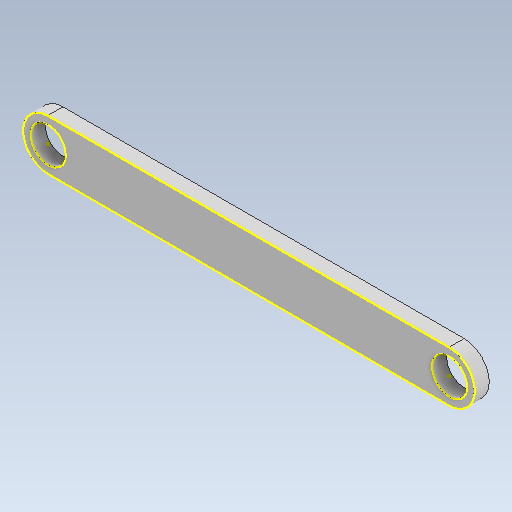
# Autodesk Inventor part: adjustable_80
Saved by Autodesk Inventor 2023 (Build 270158000, 158)
## iProperties
Created: 2023-04-16
Part Number: adjustable_80
Material: 一般
Document SubType Name: Modeling
Designer: JOU
Density: 1 g/cm^3
Appearance: 預設
Author: JOU
Autodesk Inventor part; units mm, degrees
ref_plane "YZ Plane" through (0, 0, 0) normal (1, 0, 0) x (0, 1, 0)
ref_plane "XZ Plane" through (0, 0, 0) normal (0, 1, 0) x (-1, 0, 0)
ref_plane "XY Plane" through (0, 0, 0) normal (0, 0, 1) x (1, 0, 0)
sketch "草圖1" plane through (0, 0, 0) normal (0, 0, 1) x (1, 0, 0)
  line L0 (-80, 0) -> (0, 0) construction
  line L1 (-80, -5) -> (0, -5)
  line L2 (0, 5) -> (-80, 5)
  arc A0 (-80, 5) -> (-80, -5) centre (-80, 0) ccw
  arc A1 (0, -5) -> (0, 5) centre (0, 0) ccw
  circle A2 centre (-80, 0) radius 3.5
  circle A3 centre (0, 0) radius 3.5
  point P0 (-40, 0)
  dimension "d0" = 80
  dimension "d1" = 10
  dimension "d2" = 7
  dimension "d3" = 7
  constraints: 8 end point, 4 centre point, 4 point on circle, 4 tangent, 3 coincident, 1 horizontal, 1 midpoint, 1 parallel
  measures "d0" distance of L2.start L2.end
  measures "d1" distance between parallel lines of L1 L2
  measures "d2" diameter of A2
  measures "d3" diameter of A3
extrude "擠出1" add sketch "草圖1" along normal blind 3
sketch "草圖5" plane through (0, 0, 3) normal (0, 0, 1) x (1, 0, 0)
  arc A0 (0, -5) -> (0, 5) centre (0, 0) ccw projected
  line L0 (0, 5) -> (-80, 5) projected
  arc A1 (-80, 5) -> (-80, -5) centre (-80, 0) ccw projected
  line L1 (-80, -5) -> (0, -5) projected
  circle A2 centre (0, 0) radius 3.5 projected
  circle A3 centre (-80, 0) radius 3.5 projected
